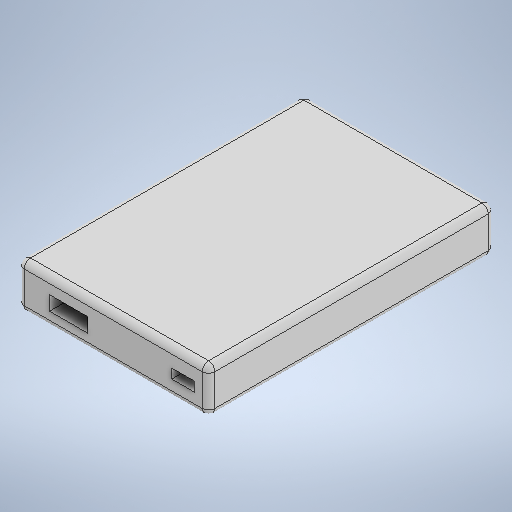
# Autodesk Inventor part: powerBank
Saved by Autodesk Inventor 2025.2 (Build 292293000, 293)
## iProperties
Created: 2026-03-17
Part Number: powerBank
Material: Genérico
Document SubType Name: Modeling
Designer: Periscopio
Density: 1 g/cm^3
Appearance: Valor por defecto
Author: Periscopio
Autodesk Inventor part; units mm, degrees
ref_plane "YZ Plane" through (0, 0, 0) normal (1, 0, 0) x (0, 1, 0)
ref_plane "XZ Plane" through (0, 0, 0) normal (0, 1, 0) x (-1, 0, 0)
ref_plane "XY Plane" through (0, 0, 0) normal (0, 0, 1) x (1, 0, 0)
sketch "Boceto1" plane through (0, 0, 0) normal (0, 1, 0) x (-1, 0, 0)
  line L0 (30, -45) -> (30, 45)
  line L1 (30, 45) -> (-30, 45)
  line L2 (-30, 45) -> (-30, -45)
  line L3 (-30, -45) -> (30, -45)
  line L4 (30, -45) -> (-30, 45) construction
  line L5 (30, 45) -> (-30, -45) construction
  point P0 (0, 0)
  dimension "d0" = 90
  dimension "d1" = 60
  constraints: 12 end point, 2 midpoint, 2 parallel, 1 perpendicular, 1 vertical
  measures "d0" distance of L0.start L0.end
  measures "d1" distance of L1.end L0.end
extrude "Extrusión1" add sketch "Boceto1" along normal blind 14
fillet "Empalme1" radius 2 1 edges at (-30, 14, 0)
fillet "Empalme2" radius 2 1 edges at (-30, 0, 0)
fillet "Empalme3" radius 2 14 edges at (-29.4142, 13.4142, 45) (-30, 7, 45) (-29.4142, 0.5858, 45) (1, 0, 45) (1, 14, 45) (30, 14, 0) (30, 7, 45) (30, 0, 0) (-29.4142, 13.4142, -45) (-30, 7, -45) (-29.4142, 0.5858, -45) (1, 0, -45) (1, 14, -45) (30, 7, -45)
sketch "Boceto3" plane through (-30, 2, 43) normal (-1, 0, 0) x (0, 0, 1)
  line L0 (-5.5242, 6.8426) -> (-12.893, 6.8426)
  line L1 (-12.893, 6.8426) -> (-12.893, 2.1055)
  line L2 (-12.893, 2.1055) -> (-5.5242, 2.1055)
  line L3 (-5.5242, 2.1055) -> (-5.5242, 6.8426)
  constraints: 8 end point, 2 parallel, 1 horizontal, 1 perpendicular
extrude "Extrusión3" add sketch "Boceto3" along normal blind 0.15
sketch "Boceto4" plane through (-28, 2, 45) normal (0, 0, 1) x (1, 0, 0)
  line L0 (-2, 0) -> (-2, 10) projected
  line L1 (56, 10) -> (0, 10) projected
  line L2 (56, -2) -> (0, -2) projected
  line L3 (8, 7) -> (20, 7)
  line L4 (20, 7) -> (20, 2.5)
  line L5 (20, 2.5) -> (8, 2.5)
  line L6 (8, 2.5) -> (8, 7)
  point P0 (28, -2)
  point P1 (14, 7)
  dimension "d14" = 4.5
  dimension "d15" = 3
  dimension "d16" = 12
  constraints: 8 end point, 2 parallel, 1 horizontal, 1 midpoint, 1 perpendicular
  measures "d14" distance of L3.end L4.end
  measures "d15" distance from line of L1 point (14, 7)
  measures "d16" distance of L4.end L5.end
extrude "Extrusión4" cut sketch "Boceto4" against normal blind 10
sketch "Boceto7" plane through (-28, 2, 45) normal (0, 0, 1) x (1, 0, 0)
  line L0 (46.4201, 6.2362) -> (53.5433, 6.2362)
  line L1 (53.5433, 6.2362) -> (53.5433, 3.2311)
  line L2 (53.5433, 3.2311) -> (46.4201, 3.2311)
  line L3 (46.4201, 3.2311) -> (46.4201, 6.2362)
  point P0 (28, -2)
  constraints: 8 end point, 2 parallel, 1 horizontal, 1 perpendicular
extrude "Extrusión5" cut sketch "Boceto7" against normal blind 10
